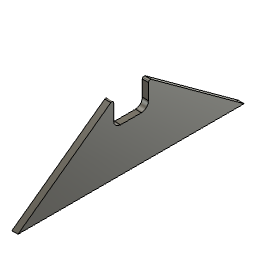
Supports (Autodesk Fusion 360 design; units mm, degrees)
Autodesk Fusion 360 part; units mm, degrees
sketch "Sketch1" plane through (0, 0, 0) normal (1, 0, 0) x (0, 0, -1)
  line L0 (10, -1.9638) -> (10, -11)
  line L1 (6, -15) -> (-6, -15)
  line L2 (-10, -11) -> (-10, -1.9638)
  line L3 (-65, -40) -> (65, -40)
  line L4 (-11.5882, -1.155) -> (-65, -40)
  line L5 (65, -40) -> (11.5882, -1.155)
  arc A0 (-10, -11) -> (-6, -15) centre (-6, -11) ccw
  arc A1 (6, -15) -> (10, -11) centre (6, -11) ccw
  arc A2 (-10, -1.9638) -> (-11.5882, -1.155) centre (-11, -1.9638) ccw
  arc A3 (11.5882, -1.155) -> (10, -1.9638) centre (11, -1.9638) ccw
  point P0 (10, 0)
  dimension "d136" = 20
  dimension "d137" = 10
  dimension "d138" = 65
  dimension "d139" = 4
  dimension "d140" = 4
  dimension "d141" = 1
  dimension "d142" = 1
  constraint vertical L0
  constraint horizontal L1
  constraint vertical L2
  constraint horizontal L3
  constraint tangent L2 A0
  constraint tangent L1 A0
  constraint tangent L0 A1
  constraint tangent L1 A1
  constraint tangent L2 A2
  constraint tangent L4 A2
  constraint coincident P0 L0
  constraint coincident P0 L5
  constraint tangent L0 A3
  constraint tangent L5 A3
  measures "d136" distance of P0 L2
  measures "d137" distance of origin P0
  measures "d138" horizontal distance of origin L3.end
  measures "d139" radius of A0
  measures "d140" radius of A1
  measures "d141" radius of A2
  measures "d142" radius of A3
extrude "Extrude1" add sketch "Sketch1" along normal blind 3.5
equation "d138 = ( 130 / 2 ) * 1 mm"
